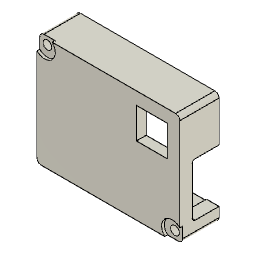
Top_PCB_Cover v1 (Autodesk Fusion 360 design; units mm, degrees)
Autodesk Fusion 360 part; units mm, degrees
sketch "Sketch1" plane through (0, 0, 0) normal (0, 1, 0) x (1, 0, 0)
  line L0 (0, 0) -> (41, 0) construction
  line L1 (41, 0) -> (41, -30) construction
  line L2 (41, -30) -> (0, -30) construction
  line L3 (0, -30) -> (0, 0) construction
  line L4 (-0.5, 0.5) -> (41.5, 0.5)
  line L5 (41.5, 0.5) -> (41.5, -30.5)
  line L6 (41.5, -30.5) -> (-0.5, -30.5)
  line L7 (-0.5, -30.5) -> (-0.5, 0.5)
  line L8 (-5, 5) -> (46, 5)
  line L9 (46, 5) -> (46, -35)
  line L10 (46, -35) -> (-5, -35)
  line L11 (-5, -35) -> (-5, 5)
  line L12 (30.5, -30.5) -> (30.5, -19.5)
  line L13 (30.5, -19.5) -> (41.5, -19.5)
  circle A0 centre (43.3031, 2.3031) radius 1.55
  circle A1 centre (-2.3031, -32.3031) radius 1.55
  circle A2 centre (-2.3031, -32.3031) radius 3.814
  circle A3 centre (43.3031, 2.3031) radius 3.814
  dimension "d1" = 41
  dimension "d2" = 30
  dimension "d3" = -0.5
  dimension "d4" = -5
  dimension "d5" = 11
  dimension "d6" = 11
  dimension "d7" = 3.1
  dimension "d8" = 3.1
  dimension "d22" = 2.55
  dimension "d23" = 2.55
  dimension "d30" = 7.6279
  dimension "d32" = 3.814
  dimension "d33" = 7.6279
  constraint horizontal L0
  constraint vertical L1
  constraint horizontal L2
  constraint vertical L3
  constraint coincident L0.start L3.end
  constraint coincident L6 L12.start
  constraint perpendicular L2 L12
  constraint coincident L5 L13.end
  constraint perpendicular L5 L13
  constraint concentric A1 A2
  constraint concentric A0 A3
  measures "d1" distance of L0.start L0.end
  measures "d2" distance of L0.start L2.end
  measures "d5" distance of L5 L12
  measures "d6" distance of L6 L13
  measures "d7" diameter of A0
  measures "d8" diameter of A1
  measures "d22" distance of L4.end A0.centre
  measures "d23" distance of L6.end A1.centre
  measures "d30" diameter of A2
  measures "d32" distance of L8.end A0.centre
  measures "d33" diameter of A3
extrude "Extrude1" add sketch "Sketch1" along normal blind 3.5 contours L4 L5 L6 L7 L12 L13 A2 A3 | L4 L5 A3 | L6 L7 A2
extrude "Extrude2" add sketch "Sketch1" along normal blind 14 contours L4 L7 L8 L11 A2 A3 | L4 L5 L8 L9 A3 | L6 L7 L10 L11 A2 | L5 L6 L9 L10 A2 A3
fillet "Fillet1" radius 1.5 4 edges at (46, 7, -5) (46, 7, 35) (-5, 7, -5) (-5, 7, 35)
ref_plane "WorkPlane1" through (20.5, 14, 15) normal (0, 1, 0) x (1, 0, 0)
sketch "Sketch2" plane through (0, 14, 0) normal (0, 1, 0) x (1, 0, 0)
  line L0 (41, -30) -> (0, -30)
  line L1 (41, 0) -> (41, -30)
  line L2 (41.5, 0.5) -> (41.5, -30.5)
  line L3 (41.5, -30.5) -> (-0.5, -30.5)
  line L4 (0, -30) -> (0, 0)
  line L5 (-0.5, -30.5) -> (-0.5, 0.5)
  line L6 (0, 0) -> (41, 0)
  line L7 (-0.5, 0.5) -> (41.5, 0.5)
  line L8 (-5, 5) -> (46, 5)
  line L9 (46, 5) -> (46, -35)
  line L10 (-5, -35) -> (-5, 5)
  line L11 (46, -35) -> (-5, -35)
  circle A0 centre (43.3031, 2.3031) radius 1.55
  circle A1 centre (-2.3031, -32.3031) radius 1.55
  line L12 (46, 0) -> (41.5, 0)
  line L13 (41.5, 0) -> (41.5, -19)
  line L14 (41.5, -19) -> (46, -19)
  line L15 (46, -19) -> (46, 0)
  line L16 (-0.5, 0) -> (-5, 0)
  line L17 (-5, 0) -> (-5, -19)
  line L18 (-5, -19) -> (-0.5, -19)
  line L19 (-0.5, -19) -> (-0.5, 0)
  line L20 (-5, 5) -> (13, 5)
  line L21 (13, 5) -> (13, 0)
  line L22 (13, 0) -> (-5, 0)
  line L23 (-5, 0) -> (-5, 5)
  line L24 (-0.5, -30.5) -> (-5, -30.5)
  line L25 (-5, -30.5) -> (-5, -27.5)
  line L26 (-5, -27.5) -> (-0.5, -27.5)
  line L27 (-0.5, -27.5) -> (-0.5, -30.5)
  dimension "d16" = 19
  dimension "d17" = 19
  dimension "d18" = 18
  dimension "d19" = 5
  dimension "d28" = 34.6062
  dimension "d29" = 45.6062
  dimension "d36" = 3
  constraint horizontal L12
  constraint vertical L13
  constraint horizontal L14
  constraint vertical L15
  constraint coincident L9 L12.start
  constraint horizontal L16
  constraint vertical L17
  constraint horizontal L18
  constraint vertical L19
  constraint coincident L5 L16.start
  constraint horizontal L20
  constraint vertical L21
  constraint horizontal L22
  constraint vertical L23
  constraint coincident L8.start L10.end
  constraint horizontal L24
  constraint vertical L25
  constraint horizontal L26
  constraint vertical L27
  constraint coincident L3.end L5.start
  measures "d16" distance of L12.start L14.end
  measures "d17" distance of L16.start L18.end
  measures "d18" distance of L8.start L20.end
  measures "d19" distance of L8.start L16.end
  measures "d28" vertical distance of A0.centre A1.centre
  measures "d29" horizontal distance of A0.centre A1.centre
  measures "d36" distance of L3.end L26.end
extrude "Extrude3" cut sketch "Sketch2" against normal blind 9.5 contours L5 L7 L8 L10 L16 L20 L21 L22 L23 | L5 L10 L16 L17 L18 L19 L22 | L5 L10 L18 L26 | L2 L9 L12 L13 L14 L15
extrude "Extrude4" cut sketch "Sketch1" along normal blind 1 contours L4 L5 L8 L9 A3 | L4 L5 A3 | L6 L7 A2 | L6 L7 L10 L11 A2 | L8 A3 | L11 A2 | L9 A3 | L10 A2
fillet "Fillet3" radius 1 4 edges at (-2.75, 4.5, 27.5) (13, 4.5, -2.75) (43.75, 4.5, 19) (43.75, 4.5, 0)
equation "d6 = d5"
equation "d9 = TOTAL_HEIGHT - WIRE_HEIGHT - 1 mm"
equation "d11 = TOTAL_HEIGHT"
equation "d20 = -WIRE_HEIGHT"
equation "d22 = d7 / 2 + 1 mm"
equation "d23 = d8 / 2 + 1 mm"
equation "TOTAL_HEIGHT = 14 mm"
equation "WIRE_HEIGHT = 9.5 mm"
equation "d30 = d33"
equation "d33 = d32 * 2"
